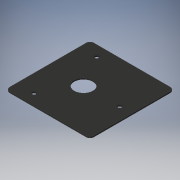
# Autodesk Inventor part: borracha isolamento respirador
Saved by Autodesk Inventor 2019.4 (Build 234330000, 330)
## iProperties
Created: 2021-02-09
Part Number: borracha isolamento respirador
Material: Borracha
Document SubType Name: Modeling
Designer: Lattes
Density: 0.93 g/cm^3
Appearance: Borracha - Preta
Author: Lattes
Autodesk Inventor part; units mm, degrees
ref_plane "YZ Plane" through (0, 0, 0) normal (1, 0, 0) x (0, 1, 0)
ref_plane "XZ Plane" through (0, 0, 0) normal (0, 1, 0) x (-1, 0, 0)
ref_plane "XY Plane" through (0, 0, 0) normal (0, 0, 1) x (1, 0, 0)
sketch "Esboço1" plane through (0, 0, 0) normal (0, 1, 0) x (-1, 0, 0)
  line L0 (0, 5) -> (-5, 5)
  line L1 (60, -55) -> (60, -60)
  line L2 (60, -60) -> (-5, -60)
  line L3 (-5, -60) -> (-5, 5)
  line L4 (-5, 5) -> (60, 5)
  line L5 (60, 5) -> (60, -60)
  line L6 (27.5, 5) -> (32.5, 5)
  circle A0 centre (32.5, -27.5) radius 7.25
  dimension "d11" = 5
  dimension "d13" = 5
  dimension "d16" = 5
  dimension "d17" = 14.5
  constraints: 14 end point, 2 parallel, 1 centre point, 1 horizontal, 1 midpoint, 1 perpendicular, 1 point on line
  measures "d11" distance of L0.start L0.end
  measures "d13" distance of L1.start L1.end
  measures "d16" distance of L6.start L6.end
  measures "d17" diameter of A0
extrude "Extrusão4" add sketch "Esboço1" along normal blind 1
sketch "Esboço2" plane through (0, 1, 0) normal (0, 1, 0) x (1, 0, 0)
  circle A0 centre (-32.5, 27.5) radius 7.25 projected
  circle A1 centre (-4.5, 27.5) radius 1.5
  point P0 (0, 0)
  dimension "d21" = 3
  constraints: 1 centre point
  measures "d21" diameter of A1
extrude "Extrusão5" cut sketch "Esboço2" against normal blind 10 contours A1
pattern_circular "Padrão circular1" count 3 over 360 about axis through (-32.5, 0, -27.5) along (0, 1, 0) of "Extrusão5"
sketch "Esboço3" plane through (-60, 0, 5) normal (0, 0, 1) x (1, 0, 0)
  line L0 (65, 0) -> (0, 0) projected
  line L1 (65, 1) -> (0, 1)
  line L2 (0, 1) -> (0, 0)
  line L3 (0, 0) -> (65, 0)
  line L4 (65, 0) -> (65, 1)
  point P0 (60, 0)
  constraints: 8 end point, 2 parallel, 1 horizontal, 1 perpendicular
sketch "Esboço4" plane through (5, 0, -60) normal (0, 0, -1) x (-1, 0, 0)
  line L0 (0, 1) -> (65, 1) projected
  line L1 (65, 1) -> (0, 1)
  line L2 (0, 1) -> (0, 0)
  line L3 (0, 0) -> (65, 0)
  line L4 (65, 0) -> (65, 1)
  point P0 (5, 0)
  constraints: 8 end point, 2 parallel, 1 horizontal, 1 perpendicular
fillet "Arredondamento1" radius 3 4 edges at (5, 0.5, -60) (5, 0.5, 5) (-60, 0.5, -60) (-60, 0.5, 5)
